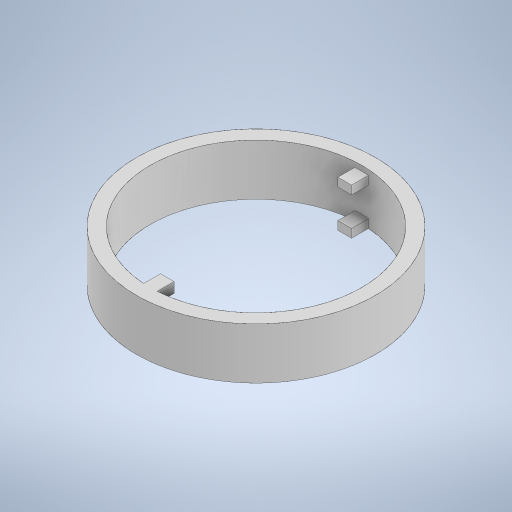
# Autodesk Inventor part: Forearm Attachment
Saved by Autodesk Inventor 2023 (Build 270158000, 158)
## iProperties
Created: 2023-04-13
Part Number: Forearm Attachment
Material: Generic
Document SubType Name: Modeling
Designer: 1senadi
Density: 1 g/cm^3
Appearance: Default
Author: 1senadi
Autodesk Inventor part; units mm, degrees
ref_plane "YZ Plane" through (0, 0, 0) normal (1, 0, 0) x (0, 1, 0)
ref_plane "XZ Plane" through (0, 0, 0) normal (0, 1, 0) x (-1, 0, 0)
ref_plane "XY Plane" through (0, 0, 0) normal (0, 0, 1) x (1, 0, 0)
sketch "Sketch1" plane through (0, 0, 0) normal (0, 1, 0) x (-1, 0, 0)
  circle A0 centre (0, 0) radius 31
  circle A1 centre (0, 0) radius 35
  line L0 (0, 31) -> (0, 26)
  line L1 (0, 26) -> (2, 26)
  line L2 (2, 26) -> (2, 30.9354)
  line L3 (0, 26) -> (-2, 26)
  line L4 (-2, 26) -> (-2, 30.9354)
  line L5 (0, -31) -> (0, -26)
  line L6 (0, -26) -> (2, -26)
  line L7 (2, -26) -> (2, -30.9354)
  line L8 (0, -26) -> (-2, -26)
  line L9 (-2, -26) -> (-2, -30.9354)
  dimension "d0" = 62
  dimension "d1" = 70
  dimension "d4" = 5
  dimension "d5" = 2
  dimension "d6" = 2
  dimension "d7" = 5
  dimension "d8" = 2
  dimension "d9" = 2
  constraints: 20 end point, 6 point on circle, 4 point on line, 3 perpendicular, 2 centre point, 2 coincident, 2 vertical, 1 parallel
  measures "d0" diameter of A0
  measures "d1" diameter of A1
  measures "d4" distance of L0.start L0.end
  measures "d5" distance of L0.end L1.end
  measures "d6" distance of L0.end L3.end
  measures "d7" distance of L5.start L5.end
  measures "d8" distance of L5.end L6.end
  measures "d9" distance of L5.end L8.end
extrude "Extrusion1" add sketch "Sketch1" along normal blind 15 contours L2 L1 L0 A0 | L0 L3 L4 A0 | A1
sketch "Sketch3" plane through (0, 0, 0) normal (0, -1, 0) x (1, 0, 0)
  arc A0 (-2, 30.9354) -> (2, 30.9354) centre (0, 0) ccw projected
  line L0 (0, -31) -> (0, -26)
  line L1 (0, -26) -> (2, -26)
  line L2 (2, -26) -> (2, -30.9354)
  line L3 (0, -26) -> (-2, -26)
  line L4 (-2, -26) -> (-2, -31)
  line L5 (31, 0) -> (-31, 0)
  line L6 (0, 31) -> (0, 26)
  line L7 (0, 26) -> (2, 26)
  line L8 (2, 26) -> (2, 30.9354)
  line L9 (0, 26) -> (-2, 26)
  line L10 (-2, 26) -> (-2, 31)
  point P0 (-2, -30.9354)
  dimension "d14" = 5
  dimension "d15" = 2
  dimension "d16" = 2
  constraints: 22 end point, 6 symmetric about line, 4 point on circle, 3 perpendicular, 2 horizontal, 1 vertical
  measures "d14" distance of L0.start L0.end
  measures "d15" distance of L0.end L1.end
  measures "d16" distance of L0.end L3.end
extrude "Extrusion3" add sketch "Sketch3" against normal blind 13.5 contours L4 L3 L0 A0 | L0 L1 L2 A0
sketch "Sketch4" plane through (-2, 0, -26) normal (0, 0, 1) x (1, 0, 0)
  line L0 (0, 0) -> (0, 13.5) projected
  line L1 (0, 6.75) -> (4, 6.75)
  line L2 (4, 0) -> (4, 13.5) projected
  line L3 (0, 6.75) -> (0, 11)
  line L4 (0, 13.5) -> (4, 13.5) projected
  line L5 (0, 11) -> (4, 11)
  line L6 (4, 11) -> (4, 6.75)
  line L7 (0, 6.75) -> (0, 2.5)
  line L8 (0, 0) -> (0, 13.5) projected
  line L9 (0, 2.5) -> (4, 2.5)
  line L10 (4, 2.5) -> (4, 6.75)
  point P0 (2, 0)
  dimension "d19" = 4.25
  dimension "d20" = 4.25
  constraints: 14 end point, 5 perpendicular, 2 midpoint, 2 point on line
  measures "d19" distance of L1.start L3.end
  measures "d20" distance of L1.start L7.end
extrude "Extrusion4" cut sketch "Sketch4" against normal up to surface contours L0 L1 L2 L9 | L0 L5 L2 L1 round surface about axis through (0, 0, 0) along (0, 1, 0) radius 31 far side no
sketch "Sketch5" plane through (2, 0, 26) normal (0, 0, -1) x (-1, 0, 0)
  line L0 (2, 0) -> (2, 15)
  line L1 (0, 15) -> (4, 15) projected
  line L2 (2, 7.5) -> (4, 7.5)
  line L3 (4, 7.5) -> (2, 7.5)
  line L4 (0, 0) -> (0, 15) projected
  line L5 (0, 7.5) -> (2, 7.5)
  line L6 (0, 7.5) -> (0, 12)
  line L7 (0, 0) -> (0, 15) projected
  line L8 (0, 12) -> (4, 12)
  line L9 (4, 0) -> (4, 15) projected
  line L10 (4, 7.5) -> (4, 12)
  line L11 (4, 7.5) -> (4, 3)
  line L12 (4, 3) -> (0, 3)
  line L13 (0, 3) -> (0, 7.5)
  point P0 (0, 12)
  point P1 (0, 3)
  dimension "d23" = 4.5
  dimension "d24" = 4.5
  constraints: 20 end point, 5 perpendicular, 4 point on line, 3 midpoint, 1 collinear, 1 horizontal
  measures "d23" distance of L5.start L6.end
  measures "d24" distance of L2.end L11.end
extrude "Extrusion5" cut sketch "Sketch5" against normal up to surface contours L12 L4 L5 L0 | L0 L2 L9 L12 | L5 L4 L8 L0 | L0 L8 L9 L2 round surface about axis through (0, 0, 0) along (0, 1, 0) radius 31 far side no
body "Solid1"
